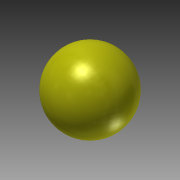
# Autodesk Inventor part: LightBulb_MaxSize
Saved by Autodesk Inventor 2014 SP1 (Build 180222100, 222)
## iProperties
Created: 2015-04-12
Part Number: LightBulb_MaxSize
Material: Rubber
Document SubType Name: Modeling
Designer: david
Density: 0.373295 g/cm^3
Appearance: Rubber - Black - Version 1.1
Mass: 58 g
Surface Area: 139.766 cm^2
Volume: 155.373 cm^3
Author: david
Autodesk Inventor part; units mm, degrees
ref_plane "YZ Plane" through (0, 0, 0) normal (1, 0, 0) x (0, 1, 0)
ref_plane "XZ Plane" through (0, 0, 0) normal (0, 1, 0) x (-1, 0, 0)
ref_plane "XY Plane" through (0, 0, 0) normal (0, 0, 1) x (1, 0, 0)
sketch "Sketch1" plane through (0, 0, 0) normal (0, 1, 0) x (-1, 0, 0)
  circle A0 centre (0, 0) radius 33.35
  line L0 (33.1749, -3.4131) -> (-33.1749, 3.4131)
  dimension "LightBulb_MaxSize" = 66.7
  constraints: 2 end point, 2 point on circle, 1 centre point, 1 coincident, 1 midpoint
  measures "LightBulb_MaxSize" diameter of A0
revolve "Revolution1" add sketch "Sketch1" angle 360 about axis through (-33.1749, 0, -3.4131) along (0.9947494, 0, 0.1023405) picked at (-7.394, 14.2479) contours A0 L0
body "Solid1"
